Autodesk Fusion 360 part; units mm, degrees
(part 2 of 2)
sketch "Sketch5" plane through (0, 0, 10) normal (0, 0, 1) x (-1, 0, 0)
  line L0 (-68, 29.876) -> (-68, 34.876)
  line L1 (-68, 34.876) -> (-72, 34.876)
  line L2 (-72, 34.876) -> (-72, -34.876)
  line L3 (-72, -34.876) -> (-68, -34.876)
  line L4 (-68, -34.876) -> (-68, -29.876)
  line L5 (-68, -29.876) -> (-62, -29.876)
  line L6 (-62, -29.876) -> (-62, -50.876)
  line L7 (-62, -50.876) -> (-68, -50.876)
  line L8 (-68, -50.876) -> (-68, -45.876)
  line L9 (-68, -45.876) -> (-72, -45.876)
  line L10 (-72, -45.876) -> (-72, -72)
  line L11 (-72, -72) -> (-45.876, -72)
  line L12 (-45.876, -72) -> (-45.876, -68)
  line L13 (-45.876, -68) -> (-50.876, -68)
  line L14 (-50.876, -68) -> (-50.876, -62)
  line L15 (-50.876, -62) -> (-29.876, -62)
  line L16 (-29.876, -62) -> (-29.876, -68)
  line L17 (-29.876, -68) -> (-34.876, -68)
  line L18 (-34.876, -68) -> (-34.876, -72)
  line L19 (-34.876, -72) -> (34.876, -72)
  line L20 (34.876, -72) -> (34.876, -68)
  line L21 (34.876, -68) -> (29.876, -68)
  line L22 (29.876, -68) -> (29.876, -62)
  line L23 (29.876, -62) -> (50.876, -62)
  line L24 (50.876, -62) -> (50.876, -68)
  line L25 (50.876, -68) -> (45.876, -68)
  line L26 (45.876, -68) -> (45.876, -72)
  line L27 (45.876, -72) -> (72.5, -72)
  line L28 (72.5, -72) -> (72.5, -45.126)
  line L29 (72.5, -45.126) -> (77.75, -45.126)
  line L30 (77.75, -45.126) -> (77.75, -50.126)
  line L31 (77.75, -50.126) -> (82.25, -50.126)
  line L32 (82.25, -50.126) -> (82.25, -30.626)
  line L33 (82.25, -30.626) -> (77.75, -30.626)
  line L34 (77.75, -30.626) -> (77.75, -35.626)
  line L35 (77.75, -35.626) -> (72.5, -35.626)
  line L36 (72.5, -35.626) -> (72.5, 35.626)
  line L37 (72.5, 35.626) -> (77.75, 35.626)
  line L38 (77.75, 35.626) -> (77.75, 30.626)
  line L39 (77.75, 30.626) -> (82.25, 30.626)
  line L40 (82.25, 30.626) -> (82.25, 50.126)
  line L41 (82.25, 50.126) -> (77.75, 50.126)
  line L42 (77.75, 50.126) -> (77.75, 45.126)
  line L43 (77.75, 45.126) -> (72.5, 45.126)
  line L44 (72.5, 45.126) -> (72.5, 72.5)
  line L45 (72.5, 72.5) -> (45.126, 72.5)
  line L46 (45.126, 72.5) -> (45.126, 77.75)
  line L47 (45.126, 77.75) -> (50.126, 77.75)
  line L48 (50.126, 77.75) -> (50.126, 82.25)
  line L49 (50.126, 82.25) -> (30.626, 82.25)
  line L50 (30.626, 82.25) -> (30.626, 77.75)
  line L51 (30.626, 77.75) -> (35.626, 77.75)
  line L52 (35.626, 77.75) -> (35.626, 72.5)
  line L53 (35.626, 72.5) -> (-35.626, 72.5)
  line L54 (-35.626, 72.5) -> (-35.626, 77.75)
  line L55 (-35.626, 77.75) -> (-30.626, 77.75)
  line L56 (-30.626, 77.75) -> (-30.626, 82.25)
  line L57 (-30.626, 82.25) -> (-50.126, 82.25)
  line L58 (-50.126, 82.25) -> (-50.126, 77.75)
  line L59 (-50.126, 77.75) -> (-45.126, 77.75)
  line L60 (-45.126, 77.75) -> (-45.126, 72.5)
  line L61 (-45.126, 72.5) -> (-72, 72.5)
  line L62 (-72, 72.5) -> (-72, 45.876)
  line L63 (-72, 45.876) -> (-68, 45.876)
  line L64 (-68, 45.876) -> (-68, 50.876)
  line L65 (-68, 50.876) -> (-62, 50.876)
  line L66 (-62, 50.876) -> (-62, 29.876)
  line L67 (-62, 29.876) -> (-68, 29.876)
  circle A0 centre (40.376, 40.376) radius 5.25
  circle A1 centre (-40.376, -40.376) radius 5.25
  circle A2 centre (0, -40.376) radius 5.25
  circle A3 centre (40.376, 0) radius 5.25
  circle A4 centre (0, 40.376) radius 5.25
  circle A5 centre (-40.376, 0) radius 5.25
  circle A6 centre (40.376, -40.376) radius 5.25
  circle A7 centre (0, 0) radius 5.25
  circle A8 centre (-40.376, 40.376) radius 5.25
  circle A9 centre (-40.376, 40.376) radius 5
  circle A10 centre (0, 40.376) radius 5
  circle A11 centre (40.376, 40.376) radius 5
  circle A12 centre (-40.376, 0) radius 5
  circle A13 centre (0, 0) radius 5
  circle A14 centre (40.376, 0) radius 5
  circle A15 centre (-40.376, -40.376) radius 5
  circle A16 centre (0, -40.376) radius 5
  circle A17 centre (40.376, -40.376) radius 5
  dimension "d217" = 10
  dimension "d218" = 10
  dimension "d219" = 10
  dimension "d220" = 10
  dimension "d221" = 10
  dimension "d222" = 10
  dimension "d223" = 10
  dimension "d224" = 10
  dimension "d225" = 10
  constraint concentric A8 A9
  constraint concentric A4 A10
  constraint concentric A0 A11
  constraint concentric A5 A12
  constraint coincident A7.centre A13.centre
  constraint concentric A3 A14
  constraint concentric A1 A15
  constraint concentric A2 A16
  constraint concentric A6 A17
  measures "d217" diameter of A9
  measures "d218" diameter of A10
  measures "d219" diameter of A11
  measures "d220" diameter of A12
  measures "d221" diameter of A13
  measures "d222" diameter of A14
  measures "d223" diameter of A15
  measures "d224" diameter of A16
  measures "d225" diameter of A17
extrude "Extrude34" add sketch "Sketch5" against normal up to surface (10 mm away) contours A0 | A1 | A2 | A3 | A4 | A5 | A6 | A7 | A8 bodies 3 in component "Breadboard"
thread "Thread1" "ISO Metric profile 10.0 M10x1.5 6H" major diameter 10.198 minor diameter 8.526 pitch 1.5 angle 60 modelled right hand crest width 0.4094 on face at (-4.9938, 0.2492, 3.3333) from (0, 0, 10) to (0, 0, 6) crest through (-4.263, 0, 9.625) on face at (35.3822, 0.2492, 3.3333) from (40.376, 0, 10) to (40.376, 0, 6) crest through (36.113, 0, 9.625) on face at (-45.3698, 40.6252, 3.3333) from (-40.376, 40.376, 10) to (-40.376, 40.376, 6) crest through (-44.639, 40.376, 9.625) on face at (-45.3698, 0.2492, 3.3333) from (-40.376, 0, 10) to (-40.376, 0, 6) crest through (-44.639, 0, 9.625) on face at (-45.3698, -40.1268, 3.3333) from (-40.376, -40.376, 10) to (-40.376, -40.376, 6) crest through (-44.639, -40.376, 9.625) on face at (-4.9938, 40.6252, 3.3333) from (0, 40.376, 10) to (0, 40.376, 6) crest through (-4.263, 40.376, 9.625) on face at (35.3822, -40.1268, 3.3333) from (40.376, -40.376, 10) to (40.376, -40.376, 6) crest through (36.113, -40.376, 9.625) on face at (-4.9938, -40.1268, 3.3333) from (0, -40.376, 10) to (0, -40.376, 6) crest through (-4.263, -40.376, 9.625) on face at (35.3822, 40.6252, 3.3333) from (40.376, 40.376, 10) to (40.376, 40.376, 6) crest through (36.113, 40.376, 9.625) on bodies 3 in component "Breadboard"
component "Breadboard" placed x (1, 0, 0) y (0, 1, 0) z (0, 0, 1) at (0, 0, 0)
hidden bodies 4 6
named bodies: "Optical Breadboard", "Connector Slot Tolerance Test", "Pegs Tolerance Test"
